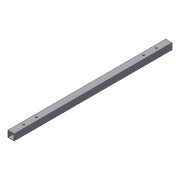
# Autodesk Inventor part: DriveTrain_SideRail
Saved by Autodesk Inventor 2012 (Build 160160000, 160)
## iProperties
Created: 2012-01-07
Part Number: DriveTrain_SideRail
Material: Aluminum-6061
Document SubType Name: Modeling
Designer: JesseK
Mass: 259.119 g
Surface Area: 1210.17 cm^2
Volume: 95.6158 cm^3
Density: 2.71 g/cm^3
Author: JesseK
Autodesk Inventor part; units mm, degrees
ref_plane "YZ Plane" through (0, 0, 0) normal (1, 0, 0) x (0, 1, 0)
ref_plane "XZ Plane" through (0, 0, 0) normal (0, 1, 0) x (-1, 0, 0)
ref_plane "XY Plane" through (0, 0, 0) normal (0, 0, 1) x (1, 0, 0)
sketch "Sketch1" plane through (0, 0, 0) normal (0, 0, 1) x (1, 0, 0)
  line L0 (0, 0) -> (25.4, 0)
  line L1 (25.4, 0) -> (25.4, 25.4)
  line L2 (25.4, 25.4) -> (0, 25.4)
  line L3 (0, 25.4) -> (0, 0)
  dimension "d0" = 25.4
  dimension "d1" = 25.4
  constraints: 8 end point, 2 parallel, 1 horizontal, 1 perpendicular
  measures "d0" distance of L2.end L0.start
  measures "d1" distance of L0.start L0.end
extrude "Extrusion1" add sketch "Sketch1" along normal blind 635
shell "Shell1" thickness 1.5875 removed faces 2 at (8.4667, 16.9333, 0) at (16.9333, 8.4667, 635)
sketch "Sketch2" plane through (0, 25.4, 0) normal (0, 1, 0) x (1, 0, 0)
  line L0 (0, -635) -> (25.4, -635) projected
  line L1 (25.4, 0) -> (0, 0) projected
  line L2 (0, 0) -> (0, -635) projected
  circle A0 centre (12.7, -50.8) radius 3.175
  circle A1 centre (12.7, -101.6) radius 3.175
  circle A2 centre (12.7, -533.4) radius 3.175
  circle A3 centre (12.7, -584.2) radius 3.175
  dimension "d7" = 50.8
  dimension "d8" = 50.8
  dimension "d9" = 12.7
  dimension "d10" = 12.7
  dimension "d11" = 6.35
  dimension "d12" = 6.35
  dimension "d13" = 12.7
  dimension "d14" = 12.7
  dimension "d15" = 50.8
  dimension "d16" = 50.8
  dimension "d17" = 6.35
  dimension "d18" = 6.35
  constraints: 4 centre point
  measures "d7" distance from line of A0.centre L1
  measures "d8" distance of A1.centre A0.centre
  measures "d9" distance from line of L2 A0.centre
  measures "d10" distance from line of L2 A1.centre
  measures "d11" diameter of A0
  measures "d12" diameter of A1
  measures "d13" distance from line of L2 A2.centre
  measures "d14" distance from line of L2 A3.centre
  measures "d15" distance from line of L0 A3.centre
  measures "d16" distance of A3.centre A2.centre
  measures "d17" diameter of A2
  measures "d18" diameter of A3
extrude "Extrusion2" cut sketch "Sketch2" against normal through all
body "Solid1"
